Autodesk Fusion 360 part; units mm, degrees
(part 2 of 2)
sketch "Sketch2" plane through (0, 34.75, 0) normal (0, 1, 0) x (1, 0, 0) in component "Gridfinity bin 5x2x5"
  line L0 (78.7214, -0.6441) -> (76.7214, -0.6441)
  line L1 (76.7214, -0.6441) -> (76.7214, -23.2816)
  spline S0 degree 5 poles (76.7214, -23.2816) (76.828, -23.4303) (77.0186, -23.7419) (77.2374, -24.252) (77.4032, -25.0107) (77.3994, -26.083) (77.1879, -27.0555) (76.8719, -27.8686) (76.5817, -28.4527) (76.4167, -28.7553) knots 0 0 0 0 0 0 0.2 0.4 0.6 0.8 1 1 1 1 1 1
  line L2 (76.469, -22.9292) -> (76.9738, -23.6339)
  line L3 (76.8308, -27.9959) -> (76.0025, -29.5147)
  arc A0 (75.0887, -28.7543) -> (76.4167, -28.7553) centre (75.753, -28.3922) ccw
  spline S1 degree 5 poles (74.7214, -23.3407) (74.6197, -23.4894) (74.4386, -23.8005) (74.2337, -24.3082) (74.0855, -25.0609) (74.1069, -26.1215) (74.3254, -27.0811) (74.6403, -27.882) (74.9265, -28.4567) (75.0887, -28.7543) knots 0 0 0 0 0 0 0.2 0.4 0.6 0.8 1 1 1 1 1 1
  line L4 (74.9636, -22.9867) -> (74.4793, -23.6947)
  line L5 (74.6798, -28.0041) -> (75.4975, -29.5045)
  line L6 (74.7214, -23.3407) -> (74.7214, -0.6441)
  line L7 (74.7214, -0.6441) -> (72.7214, -0.6441)
  line L8 (72.7214, -0.6441) -> (72.7214, -23.2816)
  spline S2 degree 5 poles (72.7214, -23.2816) (72.829, -23.4317) (73.0221, -23.7467) (73.2458, -24.2631) (73.4195, -25.0323) (73.4206, -26.1179) (73.2017, -27.0981) (72.869, -27.9135) (72.5618, -28.4974) (72.3868, -28.7994) knots 0 0 0 0 0 0 0.2 0.4 0.6 0.8 1 1 1 1 1 1
  line L9 (72.469, -22.9292) -> (72.9738, -23.6339)
  line L10 (72.8204, -28.051) -> (71.9532, -29.5477)
  arc A1 (71.054, -28.7936) -> (72.3868, -28.7994) centre (71.722, -28.4296) ccw
  spline S3 degree 5 poles (70.7214, -23.3407) (70.6192, -23.4902) (70.4364, -23.8029) (70.2269, -24.3136) (70.0692, -25.0714) (70.0777, -26.1397) (70.2892, -27.1068) (70.6029, -27.9141) (70.8905, -28.4935) (71.054, -28.7936) knots 0 0 0 0 0 0 0.2 0.4 0.6 0.8 1 1 1 1 1 1
  line L11 (70.9636, -22.9867) -> (70.4793, -23.6947)
  line L12 (70.6453, -28.0433) -> (71.4627, -29.5438)
  line L13 (70.7214, -23.3407) -> (70.7214, -0.6441)
  line L14 (70.7214, -0.6441) -> (68.7214, -0.6441)
  line L15 (68.7214, -0.6441) -> (68.7214, -23.2816)
  spline S4 degree 5 poles (68.7214, -23.2816) (68.828, -23.4303) (69.0185, -23.7421) (69.2363, -24.2522) (69.3995, -25.0109) (69.3917, -26.0829) (69.1777, -27.055) (68.8608, -27.8678) (68.5705, -28.4516) (68.4055, -28.754) knots 0 0 0 0 0 0 0.2 0.4 0.6 0.8 1 1 1 1 1 1
  line L16 (68.469, -22.9292) -> (68.9738, -23.6339)
  line L17 (68.8197, -27.9946) -> (67.9914, -29.5134)
  arc A2 (67.0886, -28.7539) -> (68.4055, -28.754) centre (67.7471, -28.3949) ccw
  spline S5 degree 5 poles (66.7214, -23.3407) (66.6197, -23.4894) (66.4386, -23.8005) (66.2338, -24.3081) (66.0856, -25.0608) (66.1069, -26.1213) (66.3253, -27.0808) (66.6402, -27.8816) (66.9264, -28.4563) (67.0886, -28.7539) knots 0 0 0 0 0 0 0.2 0.4 0.6 0.8 1 1 1 1 1 1
  line L18 (66.9636, -22.9867) -> (66.4793, -23.6947)
  line L19 (66.6797, -28.0037) -> (67.4974, -29.504)
  line L20 (66.7214, -23.3407) -> (66.7214, -0.6441)
  line L21 (66.7214, -0.6441) -> (64.7214, -0.6441)
  line L22 (64.7214, -0.6441) -> (64.7214, -23.2816)
  spline S6 degree 5 poles (64.7214, -23.2816) (64.8281, -23.4305) (65.0186, -23.7426) (65.2354, -24.2531) (65.3961, -25.0122) (65.3842, -26.0846) (65.1671, -27.0569) (64.8488, -27.8697) (64.5579, -28.4535) (64.3928, -28.7559) knots 0 0 0 0 0 0 0.2 0.4 0.6 0.8 1 1 1 1 1 1
  line L23 (64.469, -22.9292) -> (64.9738, -23.6339)
  line L24 (64.8073, -27.9967) -> (63.9782, -29.5151)
  arc A3 (63.0886, -28.7539) -> (64.3928, -28.7559) centre (63.7412, -28.3981) ccw
  spline S7 degree 5 poles (62.7214, -23.3407) (62.6197, -23.4894) (62.4386, -23.8005) (62.2338, -24.3081) (62.0856, -25.0608) (62.1069, -26.1213) (62.3253, -27.0808) (62.6402, -27.8816) (62.9264, -28.4563) (63.0886, -28.7539) knots 0 0 0 0 0 0 0.2 0.4 0.6 0.8 1 1 1 1 1 1
  line L25 (62.9636, -22.9867) -> (62.4793, -23.6947)
  line L26 (62.6797, -28.0037) -> (63.4974, -29.504)
  line L27 (62.7214, -23.3407) -> (62.7214, -0.6441)
  line L28 (62.7214, -0.6441) -> (60.7214, -0.6441)
  line L29 (60.7214, -0.6441) -> (60.7214, -23.2816)
  spline S8 degree 5 poles (60.7214, -23.2816) (60.828, -23.4303) (61.0185, -23.7421) (61.2363, -24.2522) (61.3994, -25.0109) (61.3917, -26.0829) (61.1777, -27.055) (60.8608, -27.8678) (60.5705, -28.4516) (60.4055, -28.754) knots 0 0 0 0 0 0 0.2 0.4 0.6 0.8 1 1 1 1 1 1
  line L30 (60.469, -22.9292) -> (60.9738, -23.6339)
  line L31 (60.8197, -27.9946) -> (59.9914, -29.5134)
  arc A4 (59.0886, -28.7539) -> (60.4055, -28.754) centre (59.7471, -28.3949) ccw
  spline S9 degree 5 poles (58.7214, -23.3407) (58.6197, -23.4894) (58.4386, -23.8005) (58.2338, -24.3081) (58.0856, -25.0608) (58.1069, -26.1213) (58.3253, -27.0808) (58.6402, -27.8816) (58.9264, -28.4563) (59.0886, -28.7539) knots 0 0 0 0 0 0 0.2 0.4 0.6 0.8 1 1 1 1 1 1
  line L32 (58.9636, -22.9867) -> (58.4793, -23.6947)
  line L33 (58.6797, -28.0037) -> (59.4974, -29.504)
  line L34 (58.7214, -23.3407) -> (58.7214, -0.6441)
  line L35 (58.7214, -0.6441) -> (56.7214, -0.6441)
  line L36 (56.7214, -23.3407) -> (56.7214, -0.6441)
  spline S10 degree 5 poles (56.7214, -23.3407) (56.8231, -23.4894) (57.0043, -23.8005) (57.2091, -24.3081) (57.3573, -25.0608) (57.336, -26.1213) (57.1175, -27.0808) (56.8027, -27.8816) (56.5165, -28.4563) (56.3543, -28.7539) knots 0 0 0 0 0 0 0.2 0.4 0.6 0.8 1 1 1 1 1 1
  line L37 (56.4793, -22.9867) -> (56.9636, -23.6947)
  line L38 (56.7632, -28.0037) -> (55.9454, -29.504)
  arc A5 (55.0373, -28.754) -> (56.3543, -28.7539) centre (55.6958, -28.3949) ccw
  spline S11 degree 5 poles (54.7214, -23.2816) (54.6148, -23.4303) (54.4244, -23.7421) (54.2066, -24.2522) (54.0434, -25.0109) (54.0511, -26.0829) (54.2652, -27.0551) (54.5821, -27.8678) (54.8724, -28.4516) (55.0373, -28.754) knots 0 0 0 0 0 0 0.2 0.4 0.6 0.8 1 1 1 1 1 1
  line L39 (54.9739, -22.9292) -> (54.469, -23.6339)
  line L40 (54.6232, -27.9947) -> (55.4515, -29.5134)
  line L41 (54.7214, -0.6441) -> (54.7214, -23.2816)
  line L42 (52.7214, -0.6441) -> (54.7214, -0.6441)
  line L43 (52.7214, -23.3407) -> (52.7214, -0.6441)
  spline S12 degree 5 poles (52.7214, -23.3407) (52.8231, -23.4894) (53.0043, -23.8005) (53.2091, -24.3081) (53.3573, -25.0608) (53.336, -26.1213) (53.1175, -27.0808) (52.8027, -27.8816) (52.5165, -28.4563) (52.3543, -28.7539) knots 0 0 0 0 0 0 0.2 0.4 0.6 0.8 1 1 1 1 1 1
  line L44 (52.4793, -22.9867) -> (52.9636, -23.6947)
  line L45 (52.7632, -28.0037) -> (51.9454, -29.504)
  arc A6 (51.0501, -28.7559) -> (52.3543, -28.7539) centre (51.7016, -28.3981) ccw
  spline S13 degree 5 poles (50.7214, -23.2816) (50.6147, -23.4305) (50.4243, -23.7426) (50.2074, -24.2531) (50.0468, -25.0122) (50.0587, -26.0846) (50.2757, -27.0569) (50.5941, -27.8697) (50.885, -28.4535) (51.0501, -28.7559) knots 0 0 0 0 0 0 0.2 0.4 0.6 0.8 1 1 1 1 1 1
  line L46 (50.9739, -22.9292) -> (50.469, -23.6339)
  line L47 (50.6355, -27.9967) -> (51.4646, -29.5151)
  line L48 (50.7214, -0.6441) -> (50.7214, -23.2816)
  line L49 (48.7214, -0.6441) -> (50.7214, -0.6441)
  line L50 (48.7214, -23.3407) -> (48.7214, -0.6441)
  spline S14 degree 5 poles (48.7214, -23.3407) (48.8231, -23.4894) (49.0043, -23.8005) (49.2091, -24.3081) (49.3573, -25.0608) (49.336, -26.1213) (49.1175, -27.0808) (48.8027, -27.8816) (48.5165, -28.4563) (48.3543, -28.7539) knots 0 0 0 0 0 0 0.2 0.4 0.6 0.8 1 1 1 1 1 1
  line L51 (48.4793, -22.9867) -> (48.9636, -23.6947)
  line L52 (48.7632, -28.0037) -> (47.9454, -29.504)
  arc A7 (47.0373, -28.754) -> (48.3543, -28.7539) centre (47.6958, -28.3949) ccw
  spline S15 degree 5 poles (46.7214, -23.2816) (46.6148, -23.4303) (46.4244, -23.7421) (46.2066, -24.2522) (46.0434, -25.0109) (46.0511, -26.0829) (46.2652, -27.055) (46.582, -27.8678) (46.8724, -28.4516) (47.0373, -28.754) knots 0 0 0 0 0 0 0.2 0.4 0.6 0.8 1 1 1 1 1 1
  line L53 (46.9739, -22.9292) -> (46.469, -23.6339)
  line L54 (46.6232, -27.9946) -> (47.4515, -29.5134)
  line L55 (46.7214, -0.6441) -> (46.7214, -23.2816)
  line L56 (44.7214, -0.6441) -> (46.7214, -0.6441)
  line L57 (44.7214, -23.3407) -> (44.7214, -0.6441)
  spline S16 degree 5 poles (44.7214, -23.3407) (44.8237, -23.4902) (45.0065, -23.8029) (45.216, -24.3136) (45.3736, -25.0714) (45.3651, -26.1397) (45.1537, -27.1068) (44.84, -27.9141) (44.5523, -28.4935) (44.3888, -28.7936) knots 0 0 0 0 0 0 0.2 0.4 0.6 0.8 1 1 1 1 1 1
  line L58 (44.4793, -22.9867) -> (44.9636, -23.6947)
  line L59 (44.7976, -28.0433) -> (43.9801, -29.5438)
  arc A8 (43.056, -28.7994) -> (44.3888, -28.7936) centre (43.7208, -28.4296) ccw
  spline S17 degree 5 poles (42.7214, -23.2816) (42.6139, -23.4317) (42.4207, -23.7467) (42.197, -24.2631) (42.0234, -25.0323) (42.0222, -26.1179) (42.2412, -27.0981) (42.5738, -27.9135) (42.881, -28.4974) (43.056, -28.7994) knots 0 0 0 0 0 0 0.2 0.4 0.6 0.8 1 1 1 1 1 1
  line L60 (42.9739, -22.9292) -> (42.469, -23.6339)
  line L61 (42.6224, -28.051) -> (43.4896, -29.5477)
  line L62 (42.7214, -0.6441) -> (42.7214, -23.2816)
  line L63 (40.7214, -0.6441) -> (42.7214, -0.6441)
  line L64 (40.7214, -23.3407) -> (40.7214, -0.6441)
  spline S18 degree 5 poles (40.7214, -23.3407) (40.8231, -23.4894) (41.0043, -23.8005) (41.2091, -24.3081) (41.3573, -25.0608) (41.336, -26.1213) (41.1175, -27.0808) (40.8027, -27.8816) (40.5165, -28.4563) (40.3543, -28.7539) knots 0 0 0 0 0 0 0.2 0.4 0.6 0.8 1 1 1 1 1 1
  line L65 (40.4793, -22.9867) -> (40.9636, -23.6947)
  line L66 (40.7632, -28.0037) -> (39.9454, -29.504)
  arc A9 (39.026, -28.7554) -> (40.3543, -28.7539) centre (39.6898, -28.3928) ccw
  spline S19 degree 5 poles (38.7214, -23.2816) (38.6149, -23.4303) (38.4242, -23.7419) (38.2055, -24.252) (38.0396, -25.0107) (38.0434, -26.083) (38.2548, -27.0555) (38.5708, -27.8686) (38.861, -28.4528) (39.026, -28.7554) knots 0 0 0 0 0 0 0.2 0.4 0.6 0.8 1 1 1 1 1 1
  line L67 (38.9739, -22.9292) -> (38.469, -23.6339)
  line L68 (38.6119, -27.996) -> (39.4402, -29.5147)
  line L69 (38.7214, -0.6441) -> (38.7214, -23.2816)
  line L70 (36.7214, -0.6441) -> (38.7214, -0.6441)
  line L71 (36.7214, -23.3407) -> (36.7214, -0.6441)
  spline S20 degree 5 poles (36.7214, -23.3407) (36.8229, -23.489) (37.0052, -23.7998) (37.2167, -24.3082) (37.3814, -25.0637) (37.381, -26.1275) (37.1676, -27.0861) (36.8433, -27.8824) (36.5438, -28.4521) (36.3731, -28.7466) knots 0 0 0 0 0 0 0.2 0.4 0.6 0.8 1 1 1 1 1 1
  line L72 (36.4793, -22.9867) -> (36.9636, -23.6947)
  line L73 (36.8014, -28.0074) -> (35.9448, -29.4857)
  arc A10 (35.0201, -28.7467) -> (36.3731, -28.7466) centre (35.6966, -28.3567) ccw
  spline S21 degree 5 poles (34.7214, -23.2816) (34.6151, -23.43) (34.4235, -23.7414) (34.1991, -24.2523) (34.0197, -25.0138) (34.0069, -26.0891) (34.2162, -27.0603) (34.5428, -27.8685) (34.8466, -28.4473) (35.0201, -28.7467) knots 0 0 0 0 0 0 0.2 0.4 0.6 0.8 1 1 1 1 1 1
  line L74 (34.9738, -22.9292) -> (34.469, -23.6339)
  line L75 (34.5865, -27.9984) -> (35.4537, -29.495)
  line L76 (34.7214, -0.6441) -> (34.7214, -23.2816)
  line L77 (34.7214, -0.6441) -> (32.7214, -0.6441)
  line L78 (32.7214, -0.6441) -> (32.7214, -23.2816)
  spline S22 degree 5 poles (32.7214, -23.2816) (32.828, -23.4303) (33.0186, -23.7419) (33.2374, -24.252) (33.4032, -25.0107) (33.3994, -26.083) (33.1879, -27.0555) (32.8719, -27.8686) (32.5817, -28.4527) (32.4167, -28.7553) knots 0 0 0 0 0 0 0.2 0.4 0.6 0.8 1 1 1 1 1 1
  line L79 (32.469, -22.9292) -> (32.9738, -23.6339)
  line L80 (32.8308, -27.9959) -> (32.0025, -29.5147)
  arc A11 (31.0887, -28.7543) -> (32.4167, -28.7553) centre (31.753, -28.3922) ccw
  spline S23 degree 5 poles (30.7214, -23.3407) (30.6197, -23.4894) (30.4386, -23.8005) (30.2337, -24.3082) (30.0855, -25.0609) (30.1069, -26.1215) (30.3254, -27.0811) (30.6403, -27.882) (30.9265, -28.4567) (31.0887, -28.7543) knots 0 0 0 0 0 0 0.2 0.4 0.6 0.8 1 1 1 1 1 1
  line L81 (30.9636, -22.9867) -> (30.4793, -23.6947)
  line L82 (30.6798, -28.0041) -> (31.4975, -29.5045)
  line L83 (30.7214, -23.3407) -> (30.7214, -0.6441)
  line L84 (30.7214, -0.6441) -> (28.7214, -0.6441)
  line L85 (28.7214, -0.6441) -> (28.7214, -23.2816)
  spline S24 degree 5 poles (28.7214, -23.2816) (28.829, -23.4317) (29.0221, -23.7467) (29.2458, -24.2631) (29.4195, -25.0323) (29.4206, -26.1179) (29.2017, -27.0981) (28.869, -27.9135) (28.5618, -28.4974) (28.3868, -28.7994) knots 0 0 0 0 0 0 0.2 0.4 0.6 0.8 1 1 1 1 1 1
  line L86 (28.469, -22.9292) -> (28.9738, -23.6339)
  line L87 (28.8204, -28.051) -> (27.9532, -29.5477)
  arc A12 (27.054, -28.7936) -> (28.3868, -28.7994) centre (27.722, -28.4296) ccw
  spline S25 degree 5 poles (26.7214, -23.3407) (26.6192, -23.4902) (26.4364, -23.8029) (26.2269, -24.3136) (26.0692, -25.0714) (26.0777, -26.1397) (26.2892, -27.1068) (26.6029, -27.9141) (26.8905, -28.4935) (27.054, -28.7936) knots 0 0 0 0 0 0 0.2 0.4 0.6 0.8 1 1 1 1 1 1
  line L88 (26.9636, -22.9867) -> (26.4793, -23.6947)
  line L89 (26.6453, -28.0433) -> (27.4627, -29.5438)
  line L90 (26.7214, -23.3407) -> (26.7214, -0.6441)
  line L91 (26.7214, -0.6441) -> (24.7214, -0.6441)
  line L92 (24.7214, -0.6441) -> (24.7214, -23.2816)
  spline S26 degree 5 poles (24.7214, -23.2816) (24.828, -23.4303) (25.0185, -23.7421) (25.2363, -24.2522) (25.3995, -25.0109) (25.3917, -26.0829) (25.1777, -27.055) (24.8608, -27.8678) (24.5705, -28.4516) (24.4055, -28.754) knots 0 0 0 0 0 0 0.2 0.4 0.6 0.8 1 1 1 1 1 1
  line L93 (24.469, -22.9292) -> (24.9738, -23.6339)
  line L94 (24.8197, -27.9946) -> (23.9914, -29.5134)
  arc A13 (23.0886, -28.7539) -> (24.4055, -28.754) centre (23.7471, -28.3949) ccw
  spline S27 degree 5 poles (22.7214, -23.3407) (22.6197, -23.4894) (22.4386, -23.8005) (22.2338, -24.3081) (22.0856, -25.0608) (22.1069, -26.1213) (22.3253, -27.0808) (22.6402, -27.8816) (22.9264, -28.4563) (23.0886, -28.7539) knots 0 0 0 0 0 0 0.2 0.4 0.6 0.8 1 1 1 1 1 1
  line L95 (22.9636, -22.9867) -> (22.4793, -23.6947)
  line L96 (22.6797, -28.0037) -> (23.4974, -29.504)
  line L97 (22.7214, -23.3407) -> (22.7214, -0.6441)
  line L98 (22.7214, -0.6441) -> (20.7214, -0.6441)
  line L99 (20.7214, -0.6441) -> (20.7214, -23.2816)
  spline S28 degree 5 poles (20.7214, -23.2816) (20.8281, -23.4305) (21.0186, -23.7426) (21.2354, -24.2531) (21.3961, -25.0122) (21.3842, -26.0846) (21.1671, -27.0569) (20.8488, -27.8697) (20.5579, -28.4535) (20.3928, -28.7559) knots 0 0 0 0 0 0 0.2 0.4 0.6 0.8 1 1 1 1 1 1
  line L100 (20.469, -22.9292) -> (20.9738, -23.6339)
  line L101 (20.8073, -27.9967) -> (19.9782, -29.5151)
  arc A14 (19.0886, -28.7539) -> (20.3928, -28.7559) centre (19.7412, -28.3981) ccw
  spline S29 degree 5 poles (18.7214, -23.3407) (18.6197, -23.4894) (18.4386, -23.8005) (18.2338, -24.3081) (18.0856, -25.0608) (18.1069, -26.1213) (18.3253, -27.0808) (18.6402, -27.8816) (18.9264, -28.4563) (19.0886, -28.7539) knots 0 0 0 0 0 0 0.2 0.4 0.6 0.8 1 1 1 1 1 1
  line L102 (18.9636, -22.9867) -> (18.4793, -23.6947)
  line L103 (18.6797, -28.0037) -> (19.4974, -29.504)
  line L104 (18.7214, -23.3407) -> (18.7214, -0.6441)
  line L105 (18.7214, -0.6441) -> (16.7214, -0.6441)
  line L106 (16.7214, -0.6441) -> (16.7214, -23.2816)
  spline S30 degree 5 poles (16.7214, -23.2816) (16.828, -23.4303) (17.0185, -23.7421) (17.2363, -24.2522) (17.3994, -25.0109) (17.3917, -26.0829) (17.1777, -27.055) (16.8608, -27.8678) (16.5705, -28.4516) (16.4055, -28.754) knots 0 0 0 0 0 0 0.2 0.4 0.6 0.8 1 1 1 1 1 1
  line L107 (16.469, -22.9292) -> (16.9738, -23.6339)
  line L108 (16.8197, -27.9946) -> (15.9914, -29.5134)
  arc A15 (15.0886, -28.7539) -> (16.4055, -28.754) centre (15.7471, -28.3949) ccw
  spline S31 degree 5 poles (14.7214, -23.3407) (14.6197, -23.4894) (14.4386, -23.8005) (14.2338, -24.3081) (14.0856, -25.0608) (14.1069, -26.1213) (14.3253, -27.0808) (14.6402, -27.8816) (14.9264, -28.4563) (15.0886, -28.7539) knots 0 0 0 0 0 0 0.2 0.4 0.6 0.8 1 1 1 1 1 1
  line L109 (14.9636, -22.9867) -> (14.4793, -23.6947)
  line L110 (14.6797, -28.0037) -> (15.4974, -29.504)
  line L111 (14.7214, -23.3407) -> (14.7214, -0.6441)
  line L112 (14.7214, -0.6441) -> (12.7214, -0.6441)
  line L113 (12.7214, -23.3407) -> (12.7214, -0.6441)
  spline S32 degree 5 poles (12.7214, -23.3407) (12.8231, -23.4894) (13.0043, -23.8005) (13.2091, -24.3081) (13.3573, -25.0608) (13.336, -26.1213) (13.1175, -27.0808) (12.8027, -27.8816) (12.5165, -28.4563) (12.3543, -28.7539) knots 0 0 0 0 0 0 0.2 0.4 0.6 0.8 1 1 1 1 1 1
  line L114 (12.4793, -22.9867) -> (12.9636, -23.6947)
  line L115 (12.7632, -28.0037) -> (11.9454, -29.504)
  arc A16 (11.0373, -28.754) -> (12.3543, -28.7539) centre (11.6958, -28.3949) ccw
  spline S33 degree 5 poles (10.7214, -23.2816) (10.6148, -23.4303) (10.4244, -23.7421) (10.2066, -24.2522) (10.0434, -25.0109) (10.0511, -26.0829) (10.2652, -27.0551) (10.5821, -27.8678) (10.8724, -28.4516) (11.0373, -28.754) knots 0 0 0 0 0 0 0.2 0.4 0.6 0.8 1 1 1 1 1 1
  line L116 (10.9739, -22.9292) -> (10.469, -23.6339)
  line L117 (10.6232, -27.9947) -> (11.4515, -29.5134)
  line L118 (10.7214, -0.6441) -> (10.7214, -23.2816)
  line L119 (8.7214, -0.6441) -> (10.7214, -0.6441)
  line L120 (8.7214, -23.3407) -> (8.7214, -0.6441)
  spline S34 degree 5 poles (8.7214, -23.3407) (8.8231, -23.4894) (9.0043, -23.8005) (9.2091, -24.3081) (9.3573, -25.0608) (9.336, -26.1213) (9.1175, -27.0808) (8.8027, -27.8816) (8.5165, -28.4563) (8.3543, -28.7539) knots 0 0 0 0 0 0 0.2 0.4 0.6 0.8 1 1 1 1 1 1
  line L121 (8.4793, -22.9867) -> (8.9636, -23.6947)
  line L122 (8.7632, -28.0037) -> (7.9454, -29.504)
  arc A17 (7.0501, -28.7559) -> (8.3543, -28.7539) centre (7.7016, -28.3981) ccw
  spline S35 degree 5 poles (6.7214, -23.2816) (6.6147, -23.4305) (6.4243, -23.7426) (6.2074, -24.2531) (6.0468, -25.0122) (6.0587, -26.0846) (6.2757, -27.0569) (6.5941, -27.8697) (6.885, -28.4535) (7.0501, -28.7559) knots 0 0 0 0 0 0 0.2 0.4 0.6 0.8 1 1 1 1 1 1
  line L123 (6.9739, -22.9292) -> (6.469, -23.6339)
  line L124 (6.6355, -27.9967) -> (7.4646, -29.5151)
  line L125 (6.7214, -0.6441) -> (6.7214, -23.2816)
  line L126 (4.7214, -0.6441) -> (6.7214, -0.6441)
  line L127 (4.7214, -23.3407) -> (4.7214, -0.6441)
  spline S36 degree 5 poles (4.7214, -23.3407) (4.8231, -23.4894) (5.0043, -23.8005) (5.2091, -24.3081) (5.3573, -25.0608) (5.336, -26.1213) (5.1175, -27.0808) (4.8027, -27.8816) (4.5165, -28.4563) (4.3543, -28.7539) knots 0 0 0 0 0 0 0.2 0.4 0.6 0.8 1 1 1 1 1 1
  line L128 (4.4793, -22.9867) -> (4.9636, -23.6947)
  line L129 (4.7632, -28.0037) -> (3.9454, -29.504)
  arc A18 (3.0373, -28.754) -> (4.3543, -28.7539) centre (3.6958, -28.3949) ccw
  spline S37 degree 5 poles (2.7214, -23.2816) (2.6148, -23.4303) (2.4244, -23.7421) (2.2066, -24.2522) (2.0434, -25.0109) (2.0511, -26.0829) (2.2652, -27.055) (2.582, -27.8678) (2.8724, -28.4516) (3.0373, -28.754) knots 0 0 0 0 0 0 0.2 0.4 0.6 0.8 1 1 1 1 1 1
  line L130 (2.9739, -22.9292) -> (2.469, -23.6339)
  line L131 (2.6232, -27.9946) -> (3.4515, -29.5134)
  line L132 (2.7214, -0.6441) -> (2.7214, -23.2816)
  line L133 (2.7214, -0.6441) -> (2.7214, -0.5441)
  line L134 (80.7244, -0.5441) -> (2.7214, -0.5441)
  line L135 (80.7244, -0.5441) -> (80.7214, -23.2816)
  spline S38 degree 5 poles (80.7214, -23.2816) (80.828, -23.4303) (81.0186, -23.7419) (81.2374, -24.252) (81.4032, -25.0107) (81.3994, -26.083) (81.1879, -27.0555) (80.8719, -27.8686) (80.5817, -28.4527) (80.4167, -28.7553) knots 0 0 0 0 0 0 0.2 0.4 0.6 0.8 1 1 1 1 1 1
  line L136 (80.469, -22.9292) -> (80.9738, -23.6339)
  line L137 (80.8308, -27.9959) -> (80.0025, -29.5147)
  arc A19 (79.0887, -28.7543) -> (80.4167, -28.7553) centre (79.753, -28.3922) ccw
  spline S39 degree 5 poles (78.7214, -23.3407) (78.6197, -23.4894) (78.4386, -23.8005) (78.2337, -24.3082) (78.0855, -25.0609) (78.1069, -26.1215) (78.3254, -27.0811) (78.6403, -27.882) (78.9265, -28.4567) (79.0887, -28.7543) knots 0 0 0 0 0 0 0.2 0.4 0.6 0.8 1 1 1 1 1 1
  line L138 (78.9636, -22.9867) -> (78.4793, -23.6947)
  line L139 (78.6798, -28.0041) -> (79.4975, -29.5045)
  line L140 (78.7214, -23.3407) -> (78.7214, -0.6441)
  dimension "d478" = 0.1
  dimension "d479" = 2
  dimension "d480" = 2
  dimension "d481" = 2
  dimension "d482" = 2
  dimension "d483" = 2
  dimension "d484" = 2
  dimension "d485" = 2
  dimension "d486" = 2
  dimension "d487" = 2
  dimension "d488" = 2
  dimension "d489" = 2
  dimension "d490" = 2
  dimension "d491" = 2
  dimension "d492" = 2
  dimension "d493" = 2
  dimension "d494" = 2
  dimension "d495" = 2
  dimension "d496" = 2
  dimension "d497" = 0.1
  dimension "d498" = 0.1
  dimension "d499" = 0.1
  dimension "d500" = 0.1
  dimension "d501" = 0.1
  dimension "d502" = 0.1
  dimension "d503" = 0.1
  dimension "d504" = 0.1
  dimension "d505" = 0.1
  dimension "d506" = 0.1
  dimension "d507" = 0.1
  dimension "d508" = 0.1
  dimension "d509" = 0.1
  dimension "d510" = 0.1
  dimension "d511" = 0.1
  dimension "d512" = 0.1
  dimension "d513" = 0.1
  dimension "d514" = 0.1
  constraint tangent S0 A0
  constraint tangent A0 S1
  constraint midpoint S1.start L4
  constraint midpoint A0.start L5
  constraint midpoint L1.end L2
  constraint midpoint S0.end L3
  constraint tangent A1 S3
  constraint midpoint S3.start L11
  constraint midpoint A1.start L12
  constraint midpoint L8.end L9
  constraint midpoint S2.end L10
  constraint midpoint S5.start L18
  constraint midpoint A2.start L19
  constraint midpoint L15.end L16
  constraint midpoint S4.end L17
  constraint midpoint L22.end L23
  constraint midpoint S6.end L24
  constraint tangent A3 S7
  constraint midpoint S7.start L25
  constraint midpoint A3.start L26
  constraint tangent S8 A4
  constraint tangent A4 S9
  constraint midpoint S9.start L32
  constraint midpoint A4.start L33
  constraint midpoint L29.end L30
  constraint midpoint S8.end L31
  constraint tangent S22 A11
  constraint tangent A11 S23
  constraint midpoint S23.start L81
  constraint midpoint A11.start L82
  constraint midpoint L78.end L79
  constraint midpoint S22.end L80
  constraint tangent A12 S25
  constraint midpoint S25.start L88
  constraint midpoint A12.start L89
  constraint midpoint L85.end L86
  constraint midpoint S24.end L87
  constraint midpoint S27.start L95
  constraint midpoint A13.start L96
  constraint midpoint L92.end L93
  constraint midpoint S26.end L94
  constraint midpoint L99.end L100
  constraint midpoint S28.end L101
  constraint tangent A14 S29
  constraint midpoint S29.start L102
  constraint midpoint A14.start L103
  constraint tangent S30 A15
  constraint tangent A15 S31
  constraint midpoint S31.start L109
  constraint midpoint A15.start L110
  constraint midpoint L106.end L107
  constraint midpoint S30.end L108
  constraint horizontal L77
  constraint horizontal L134
  constraint tangent S38 A19
  constraint tangent A19 S39
  constraint midpoint S39.start L138
  constraint midpoint A19.start L139
  constraint midpoint L135.end L136
  constraint midpoint S38.end L137
  constraint perpendicular L133 L134
  measures "d478" distance of L0 L134
  measures "d479" distance of L6 L8
  measures "d480" distance of L13 L15
  measures "d481" distance of L20 L22
  measures "d482" distance of L27 L29
  measures "d483" distance of L34 L36
  measures "d484" distance of L41 L43
  measures "d485" distance of L48 L50
  measures "d486" distance of L55 L57
  measures "d487" distance of L62 L64
  measures "d488" distance of L69 L71
  measures "d489" distance of L76 L78
  measures "d490" distance of L83 L85
  measures "d491" distance of L90 L92
  measures "d492" distance of L97 L99
  measures "d493" distance of L104 L106
  measures "d494" distance of L111 L113
  measures "d495" distance of L118 L120
  measures "d496" distance of L125 L127
  measures "d498" distance of L14 L134
  measures "d500" distance of L28 L134
  measures "d501" distance of L35 L134
  measures "d502" distance of L42 L134
  measures "d503" distance of L49 L134
  measures "d504" distance of L56 L134
  measures "d505" distance of L63 L134
  measures "d506" distance of L70 L134
  measures "d507" distance of L77 L134
  measures "d508" distance of L84 L134
  measures "d509" distance of L91 L134
  measures "d510" distance of L98 L134
  measures "d511" distance of L105 L134
  measures "d512" distance of L112 L134
  measures "d513" distance of L119 L134
  measures "d514" distance of L126 L134
extrude "Extrude11" add sketch "Sketch1" along normal blind 5 bodies 11 in component "Gridfinity bin 5x2x5"
extrude "Extrude12" add sketch "Sketch2" along normal blind 5 bodies 11 in component "Gridfinity bin 5x2x5"
component "Gridfinity bin 5x2x5" placed x (1, 0, 0) y (0, 1, 0) z (0, 0, 1) at (0, 0, 0)
equation "wire_length = 140 mm"
equation "d330 = -( 2.40 mm )"
equation "d360 = -( 2.40 mm )"
equation "d370 = -( 0.60 mm )"
equation "d387 = -( 29.00 mm )"
equation "d402 = ( 207.1 mm - wire_length ) / 2"
equation "d403 = ( 207.1 mm - wire_length ) / 2"
named bodies: "Base", "Base (1)", "Base (2)", "Base (3)", "Base (4)", "Base (5)", "Base (6)", "Base (7)", "Base (8)", "Base (9)", "Gridfinity bin 5x2x5", "Lip body", "Lip cutout", "Inner cutout"
